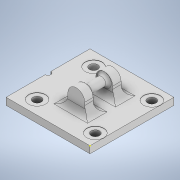
# Autodesk Inventor part: Upper mount
Saved by Autodesk Inventor 2022 (Build 260153000, 153)
## iProperties
Created: 2022-03-20
Part Number: Upper mount
Material: Generic
Document SubType Name: Modeling
Designer: Dahway
Density: 1 g/cm^3
Appearance: Default
Author: Dahway
Autodesk Inventor part; units mm, degrees
ref_plane "YZ Plane" through (0, 0, 0) normal (1, 0, 0) x (0, 1, 0)
ref_plane "XZ Plane" through (0, 0, 0) normal (0, 1, 0) x (-1, 0, 0)
ref_plane "XY Plane" through (0, 0, 0) normal (0, 0, 1) x (1, 0, 0)
sketch "Sketch1" plane through (0, 0, 0) normal (0, 1, 0) x (-1, 0, 0)
  line L0 (0, 0) -> (30, 0)
  line L1 (30, 0) -> (30, -30)
  line L2 (30, -30) -> (0, -30)
  line L3 (0, -30) -> (0, 0)
  dimension "d0" = 30
  dimension "d1" = 30
  constraints: 8 end point, 2 parallel, 1 horizontal, 1 perpendicular
  measures "d0" distance of L1.end L2.end
  measures "d1" distance of L0.end L1.end
extrude "Extrusion1" add sketch "Sketch1" along normal blind 2.5
sketch "Sketch2" plane through (0, 2.5, 0) normal (0, 1, 0) x (1, 0, 0)
  line L0 (-30, 0) -> (0, 0) projected
  line L1 (0, 0) -> (0, 30) projected
  line L2 (0, 30) -> (-30, 30) projected
  point P0 (-3, 4.9)
  point P1 (-3, 25.1)
  point P2 (-23.8, 25.1)
  point P3 (-23.8, 4.9)
  dimension "d14" = 20.2
  dimension "d15" = 20.8
  dimension "d16" = 4.9
  dimension "d17" = 20.2
  dimension "d18" = 3
  dimension "d19" = 20.8
  dimension "d20" = 4.9
  dimension "d21" = 4.9
  measures "d14" distance of point (-23.8, 25.1) point (-23.8, 4.9)
  measures "d15" distance of point (-3, 25.1) point (-23.8, 25.1)
  measures "d16" distance from line of L0 point (-3, 4.9)
  measures "d17" distance of point (-3, 25.1) point (-3, 4.9)
  measures "d18" distance from line of L1 point (-3, 4.9)
  measures "d19" distance of point (-3, 4.9) point (-23.8, 4.9)
  measures "d20" distance from line of L2 point (-3, 25.1)
  measures "d21" distance from line of L0 point (-23.8, 4.9)
hole "Hole1" at (-3, 2.5, -4.9) at (-3, 2.5, -25.1) at (-23.8, 2.5, -25.1) at (-23.8, 2.5, -4.9) direction (0, -1, 0) diameter 3 end through all counterbore diameter 6 counterbore depth 0.1
sketch "Sketch3" plane through (0, 2.5, 0) normal (0, 1, 0) x (1, 0, 0)
  line L0 (-30, 30) -> (-30, 0) projected
  circle A0 centre (-30, 15) radius 1
  point P0 (0, 0)
  point P1 (-30, 16)
  point P2 (-30, 14)
  dimension "d11" = 2
  constraints: 1 centre point, 1 midpoint
  measures "d11" diameter of A0
extrude "Extrusion2" cut sketch "Sketch3" against normal blind 1 contours A0 L0 picked at (-29.6652, 15.1995)
sketch "Sketch4" plane through (0, 2.5, 0) normal (0, 1, 0) x (1, 0, 0)
  line L0 (-10.4, 11.5) -> (-16.4, 11.5)
  line L1 (-16.4, 11.5) -> (-16.4, 8.5)
  line L2 (-16.4, 8.5) -> (-10.4, 8.5)
  line L3 (-10.4, 8.5) -> (-10.4, 11.5)
  line L4 (-30, 0) -> (0, 0) projected
  line L5 (0, 0) -> (0, 30) projected
  line L6 (-10.4, 18.5) -> (-16.4, 18.5)
  line L7 (-16.4, 18.5) -> (-16.4, 21.5)
  line L8 (-16.4, 21.5) -> (-10.4, 21.5)
  line L9 (-10.4, 21.5) -> (-10.4, 18.5)
  line L10 (-30, 30) -> (-30, 16) projected
  dimension "d22" = 6
  dimension "d23" = 3
  dimension "d24" = 8.5
  dimension "d25" = 10.4
  dimension "d26" = 3
  dimension "d27" = 7
  dimension "d28" = 13.6
  dimension "d29" = 10.4
  constraints: 16 end point, 4 parallel, 2 horizontal, 2 perpendicular
  measures "d22" distance of L2.end L1.end
  measures "d23" distance of L1.end L0.end
  measures "d24" distance between parallel lines of L4 L2
  measures "d25" distance between parallel lines of L5 L3
  measures "d26" distance of L6.end L7.end
  measures "d27" distance between parallel lines of L6 L0
  measures "d28" distance between parallel lines of L7 L10
  measures "d29" distance between parallel lines of L5 L9
extrude "Extrusion3" add sketch "Sketch4" along normal blind 7
fillet "Fillet1" radius 3 8 edges at (-10.4, 9.5, -10) (-16.4, 9.5, -10) (-16.4, 9.5, -20) (-10.4, 9.5, -20) (-10.4, 2.5, -20) (-10.4, 2.5, -10) (-16.4, 2.5, -20) (-16.4, 2.5, -10)
sketch "Sketch5" plane through (-7.4, 2.5, -11.5) normal (0, 0, -1) x (-1, 0, 0)
  circle A0 centre (6, 4.5) radius 1.5
  line L0 (12, 0) -> (0, 0) projected
  line L1 (3, 3) -> (3, 4) projected
  point P0 (-7.4, -2.5)
  dimension "d33" = 3
  dimension "d34" = 4.5
  dimension "d35" = 3
  constraints: 1 centre point
  measures "d33" diameter of A0
  measures "d34" distance from line of L0 A0.centre
  measures "d35" distance from line of L1 A0.centre
extrude "Extrusion4" add sketch "Sketch5" along normal up to surface (7 mm away)
fillet "Fillet2" radius 1 2 edges at (-11.9, 7, -11.5) (-11.9, 7, -18.5)
fillet "Fillet3" radius 2 4 edges at (-13.4, 2.5, -11.5) (-13.4, 2.5, -18.5) (-13.4, 2.5, -8.5) (-13.4, 2.5, -21.5)
sketch "Sketch6" plane through (0, 2.5, 0) normal (0, 1, 0) x (1, 0, 0)
  point P0 (0, 0)
body "Solid1"
